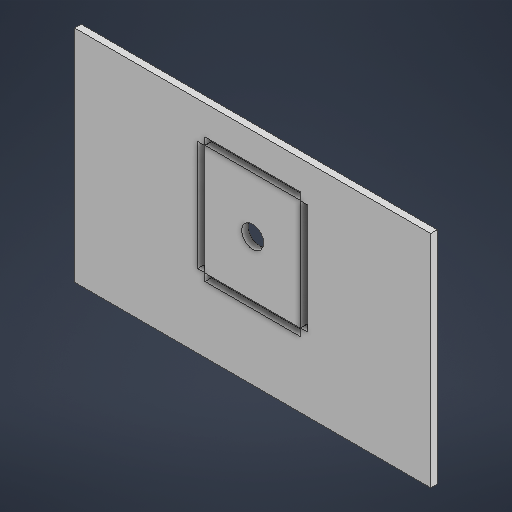
# Autodesk Inventor part: Part4
Saved by Autodesk Inventor 2026.2 (Build 302298010, 298A)
## iProperties
Created: 2026-03-02
Part Number: Part4
Material: Generic
Document SubType Name: Modeling
Designer: shahd
Density: 1 g/cm^3
Appearance: Default
Mass: 8.27591 g
Surface Area: 101.906 cm^2
Volume: 8.27591 cm^3
Author: shahd
Autodesk Inventor part; units mm, degrees
ref_plane "YZ Plane" through (0, 0, 0) normal (1, 0, 0) x (0, 1, 0)
ref_plane "XZ Plane" through (0, 0, 0) normal (0, 1, 0) x (-1, 0, 0)
ref_plane "XY Plane" through (0, 0, 0) normal (0, 0, 1) x (1, 0, 0)
sketch "Sketch1" plane through (0, 0, 0) normal (0, 0, 1) x (1, 0, 0)
  line L0 (0, 0) -> (97, 0)
  line L1 (97, 0) -> (97, 60)
  line L2 (97, 60) -> (0, 60)
  line L3 (0, 60) -> (0, 0)
  circle A0 centre (48.5, 35) radius 3
  line L4 (63.5, 50) -> (61.5, 50)
  line L5 (61.5, 50) -> (61.5, 20)
  line L6 (61.5, 20) -> (63.5, 20)
  line L7 (63.5, 20) -> (63.5, 50)
  line L8 (33.5, 50) -> (35.5, 50)
  line L9 (35.5, 50) -> (35.5, 20)
  line L10 (35.5, 20) -> (33.5, 20)
  line L11 (33.5, 20) -> (33.5, 50)
  line L12 (35.5, 52.0718) -> (61.5, 52.0718)
  line L13 (61.5, 52.0718) -> (61.5, 50.0718)
  line L14 (61.5, 50.0718) -> (35.5, 50.0718)
  line L15 (35.5, 50.0718) -> (35.5, 52.0718)
  line L16 (48.5, 35) -> (31.2053, 35)
  line L17 (31.2053, 35) -> (48.5, 35)
  line L18 (48.5, 35) -> (67.3058, 35)
  line L19 (35.5, 17.9282) -> (61.5, 17.9282)
  line L20 (61.5, 19.9282) -> (35.5, 19.9282)
  line L21 (61.5, 17.9282) -> (61.5, 19.9282)
  line L22 (35.5, 17.9282) -> (35.5, 19.9282)
  point P0 (0, 30)
  point P1 (62.5, 50)
  dimension "d2" = 97
  dimension "d3" = 60
  dimension "d4" = 6
  dimension "d6" = 25
  dimension "d7" = 48.5
  dimension "d8" = 2
  dimension "d9" = 30
  dimension "d10" = 10
  dimension "d12" = 15
  dimension "d13" = 2
  dimension "d14" = 30
  dimension "d15" = 15
  dimension "d16" = 2
  dimension "d20" = 26
  dimension "d21" = 0
  constraints: 46 end point, 9 equal length, 5 horizontal, 5 perpendicular, 4 symmetric about line, 2 midpoint, 1 centre point, 1 point on line, 1 vertical
  measures "d2" distance of L1.end L2.end
  measures "d3" distance of L0.end L1.end
  measures "d4" diameter of A0
  measures "d6" distance from line of L2 L16.start
  measures "d7" distance from line of L3 L16.start
  measures "d8" distance of L5.end L6.end
  measures "d9" distance of L4.end L5.end
  measures "d10" distance from line of point (62.5, 50) L2
  measures "d12" distance from line of L16.start L7
  measures "d13" distance of L8.start L8.end
  measures "d14" distance of L8.end L9.end
  measures "d15" distance from line of L11 L16.start
  measures "d16" distance of L12.end L13.end
  measures "d20" distance of L13.end L14.end
  measures "d21" distance between parallel lines of L9 L15
extrude "Extrusion1" add sketch "Sketch1" along normal mid plane 1.8
body "Solid1"
